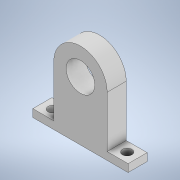
# Autodesk Inventor part: sopoetellantas
Saved by Autodesk Inventor 2021 (Build 250183000, 183)
## iProperties
Created: 2021-02-06
Part Number: sopoetellantas
Material: Genérico
Document SubType Name: Modeling
Designer: jaime
Density: 1 g/cm^3
Appearance: Valor por defecto
Author: jaime
Autodesk Inventor part; units mm, degrees
ref_plane "YZ Plane" through (0, 0, 0) normal (1, 0, 0) x (0, 1, 0)
ref_plane "XZ Plane" through (0, 0, 0) normal (0, 1, 0) x (-1, 0, 0)
ref_plane "XY Plane" through (0, 0, 0) normal (0, 0, 1) x (1, 0, 0)
sketch "Boceto1" plane through (0, 0, 0) normal (0, 0, 1) x (1, 0, 0)
  arc A0 (0, 14) -> (-14, 0) centre (0, 0) ccw
  line L0 (-14, 0) -> (-14, -26.9516)
  line L1 (-14, -26.9516) -> (-25, -26.9516)
  line L2 (-25, -26.9516) -> (-25, -30.9943)
  line L3 (-25, -30.9943) -> (0, -30.9943)
  line L4 (0, -30.9943) -> (0, 14) construction
  arc A1 (0, 7.5) -> (0, -7.5) centre (0, 0) ccw
  arc A2 (14, 0) -> (0, 14) centre (0, 0) ccw
  line L5 (14, 0) -> (14, -26.9516)
  line L6 (14, -26.9516) -> (25, -26.9516)
  line L7 (25, -26.9516) -> (25, -30.9943)
  line L8 (25, -30.9943) -> (0, -30.9943)
  arc A3 (0, -7.5) -> (0, 7.5) centre (0, 0) ccw
  dimension "d2" = 7.5
  dimension "d6" = 50
  dimension "d7" = 28
  constraints: 18 end point, 8 point on circle, 4 centre point, 4 symmetric about line, 3 coincident, 3 vertical, 2 point on line, 1 horizontal, 1 perpendicular, 1 tangent, 2 other
  measures "d2" radius of A1
  measures "d6" distance between parallel lines of L2 L7
  measures "d7" distance between parallel lines of L0 L5
extrude "Extrusión1" add sketch "Boceto1" along normal blind 10
sketch "Boceto2" plane through (-25, -26.9516, 0) normal (0, 1, 0) x (1, 0, 0)
  line L0 (11, 0) -> (39, 0) projected
  line L1 (0, -10) -> (50, -10) projected
  line L2 (11, 0) -> (0, -10)
  line L3 (11, -10) -> (39, -10) projected
  line L4 (0, 0) -> (50, 0) projected
  line L5 (11, -10) -> (0, 0)
  line L6 (0, 0) -> (50, -10)
  line L7 (0, -10) -> (50, 0)
  line L8 (25, -5) -> (25, 11.6359)
  circle A0 centre (5.5, -5) radius 2.5
  circle A1 centre (44.5, -5) radius 2.5
  point P0 (25, 0)
  dimension "d3" = 5
  constraints: 10 end point, 2 centre point, 2 midpoint, 1 symmetric about line, 1 vertical, 1 other
  measures "d3" diameter of A0
extrude "Extrusión2" cut sketch "Boceto2" against normal blind 5 contours A0 L5 L2 | L2 L5 A0 | L5 L2 A0 | L5 A0 L2 | A1
